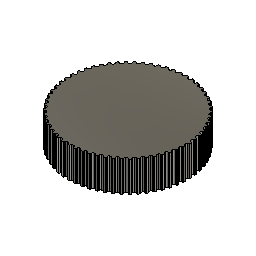
gear_62z (Autodesk Fusion 360 design; units mm, degrees)
Autodesk Fusion 360 part; units mm, degrees
sketch "Sketch1" plane through (0, 0, 0) normal (0, 0, 1) x (1, 0, 0) in component "gt2 pulley"
  circle A0 centre (0, 0) radius 19.7352 construction
  circle A1 centre (0, 0) radius 18.7312 construction
  line L0 (0, 0) -> (0, 19.7352) construction
  line L1 (0, 0) -> (0.9996, 19.7099) construction
  line L2 (0, 0) -> (1.4061, 19.6851) construction
  circle A2 centre (0, 0) radius 19.4812 construction
  arc A3 (0.3919, 19.343) -> (0.4641, 19.0491) centre (1.388, 19.4317) ccw
  circle A4 centre (0, 0) radius 19.3312 construction
  arc A5 (0.2443, 19.4797) -> (0, 19.4812) centre (0, 0) ccw
  arc A6 (0.3919, 19.343) -> (0.2443, 19.4797) centre (0.2425, 19.3297) ccw
  arc A7 (0.4641, 19.0491) -> (0.9487, 18.7072) centre (0.9768, 19.2615) ccw
  arc A8 (0, 19.4812) -> (-0.2443, 19.4797) centre (0, 0) ccw
  arc A9 (-0.2443, 19.4797) -> (-0.3919, 19.343) centre (-0.2425, 19.3297) ccw
  arc A10 (-0.4641, 19.0491) -> (-0.3919, 19.343) centre (-1.388, 19.4317) ccw
  arc A11 (-0.9486, 18.7072) -> (-0.4641, 19.0491) centre (-0.9768, 19.2615) ccw
  arc A12 (0.9487, 18.7072) -> (-0.9487, 18.7072) centre (0, 0) ccw
  point P0 (1.388, 19.4317)
  point P1 (0, 19.4812)
  dimension "d18" = 39.4704
  dimension "d19" = 2.903
  dimension "d22" = 1.004
  dimension "d24" = 0.75
  dimension "d26" = 1
  dimension "d27" = 0.15
  dimension "d28" = 0.15
  dimension "d47" = 0.555
  dimension "d52" = 3.812
  constraint coincident A0.centre A1.centre
  constraint coincident A0 L0.end
  constraint vertical L0
  constraint coincident A0 L1.end
  constraint coincident A0 L2.end
  constraint concentric A1 A2
  constraint coincident A1 A7.end
  constraint coincident L1 A7.end
  constraint coincident A2 P0
  constraint coincident L2 P0
  constraint coincident P0 A3.centre
  constraint coincident A2 P1
  constraint coincident L0 P1
  constraint concentric A2 A4
  constraint coincident P1 A5.end
  constraint coincident A4 A6.centre
  constraint coincident A3.start A6.start
  constraint tangent A3 A6
  constraint tangent A3 A7
  constraint symmetric L0 A7.end A12.end
  constraint symmetric L0 A3.start A9.end
  constraint symmetric L0 A3.end A10.start
  constraint symmetric L0 A3 A10
  constraint symmetric L0 A5.start A8.end
  constraint symmetric L0 P1 A5.end
  constraint symmetric L0 A5 A8
  constraint symmetric L0 A6 A9
  constraint symmetric L0 A7 A11
  constraint coincident A1 A11.start
  constraint tangent A1 A7
  constraint coincident L1 A7.centre
  measures "d18" diameter of A0
  measures "d19" angle of L0 L1
  measures "d22" distance of A0 A1
  measures "d24" distance of A1 A2
  measures "d26" radius of A3
  measures "d27" distance of A2 A4
  measures "d28" radius of A6
  measures "d47" radius of A7
extrude "Extrude1" add sketch "Sketch1" along normal blind 10 makes body 1
pattern_circular "C-Pattern1" count 62 over 360 about axis through (0, 0, 1.75) along (0, 0, 1) of bodies 1 makes body 2 at (-1.1593, 18.6953, 3.3333) makes body 3 at (-4.4904, 18.185, 6.6667) makes body 4 at (-5.7079, 17.8404, 6.6667) makes body 5 at (-6.7028, 17.4909, 3.3333) makes body 6 at (-8.9979, 16.4285, 6.6667) makes body 7 at (-10.7869, 15.3135, 6.6667) makes body 8 at (-12.7514, 13.7208, 6.6667) makes body 9 at (-13.0572, 13.4301, 3.3333) makes body 10 at (-15.2524, 10.8731, 6.6667) makes body 11 at (-16.2741, 9.2742, 6.6667) makes body 12 at (-17.1289, 7.5802, 6.6667) makes body 13 at (-17.2953, 7.1925, 3.3333) makes body 14 at (-18.3041, 3.977, 6.6667) makes body 15 at (-18.6126, 2.1048, 6.6667) makes body 16 at (-18.73, 0.211, 6.6667) makes body 17 at (-18.73, -0.2109, 6.6667) makes body 18 at (-18.3891, -3.5636, 6.6667) makes body 19 at (-18.3042, -3.9769, 3.3333) makes body 20 at (-17.6016, -6.4064, 6.6667) makes body 21 at (-17.1289, -7.5801, 6.6667) makes body 22 at (-15.4935, -10.5267, 6.6667) makes body 23 at (-14.7475, -11.5486, 6.6667) makes body 24 at (-14.0742, -12.3602, 3.3333) makes body 25 at (-12.1208, -14.2809, 6.6667) makes body 26 at (-10.0866, -15.7835, 6.6667) makes body 27 at (-8.998, -16.4285, 6.6667) makes body 28 at (-6.7029, -17.4908, 6.6667) makes body 29 at (-5.5068, -17.9034, 6.6667) makes body 30 at (-3.0449, -18.4821, 6.6667) makes body 31 at (-1.3699, -18.6811, 6.6667) makes body 32 at (-0.738, -18.7167, 3.3333) makes body 33 at (1.9998, -18.6242, 6.6667) makes body 34 at (4.4904, -18.185, 6.6667) makes body 35 at (6.1081, -17.7073, 6.6667) makes body 36 at (6.7028, -17.4909, 3.3333) makes body 37 at (8.9979, -16.4285, 6.6667) makes body 38 at (10.7869, -15.3135, 6.6667) makes body 39 at (12.7514, -13.7208, 6.6667) makes body 40 at (13.0572, -13.4301, 3.3333) makes body 41 at (14.8765, -11.382, 6.6667) makes body 42 at (15.9516, -9.8186, 6.6667) makes body 43 at (17.1289, -7.5802, 6.6667) makes body 44 at (17.6016, -6.4065, 6.6667) makes body 45 at (18.3041, -3.977, 6.6667) makes body 46 at (18.6126, -2.1048, 6.6667) makes body 47 at (18.73, -0.211, 6.6667) makes body 48 at (18.73, 0.2109, 3.3333) makes body 49 at (18.6126, 2.1047, 3.3333) makes body 50 at (18.3042, 3.9769, 3.3333) makes body 51 at (17.8079, 5.8083, 3.3333) makes body 52 at (16.7703, 8.3436, 6.6667) makes body 53 at (16.2742, 9.2741, 3.3333) makes body 54 at (14.349, 12.0401, 6.6667) makes body 55 at (14.0742, 12.3602, 3.3333) makes body 56 at (11.6316, 14.6821, 6.6667) makes body 57 at (10.6139, 15.4338, 6.6667) makes body 58 at (9.7285, 16.0067, 3.3333) makes body 59 at (7.4836, 17.1713, 6.6667) makes body 60 at (5.708, 17.8403, 6.6667) makes body 61 at (4.4906, 18.185, 3.3333) makes body 62 at (2.6278, 18.546, 3.3333)
sketch "Sketch2" plane through (0, 0, 10) normal (0, 0, 1) x (-1, 0, 0)
  arc A0 (-12.8969, -14.4214) -> (-12.8739, -14.6212) centre (-12.7748, -14.5086) ccw
  arc A1 (-12.8739, -14.6212) -> (-12.5031, -14.9395) centre (0, 0) ccw
  arc A2 (-12.5031, -14.9395) -> (-12.3021, -14.9319) centre (-12.4068, -14.8245) ccw
  arc A3 (-12.056, -14.756) -> (-12.3021, -14.9319) centre (-11.6041, -15.6481) ccw
  arc A4 (-11.4656, -14.8121) -> (-12.056, -14.756) centre (-11.8052, -15.2511) ccw
  arc A5 (-12.9052, -13.5762) -> (-11.4656, -14.8121) centre (0, 0) ccw
  arc A6 (-12.7602, -14.1514) -> (-12.9052, -13.5762) centre (-13.2876, -13.9785) ccw
  arc A7 (-12.8969, -14.4214) -> (-12.7602, -14.1514) centre (-13.7104, -13.8399) ccw
  circle A8 centre (0, 0) radius 18.7312
  constraint concentric A1 A8
extrude "Extrude2" add sketch "Sketch2" against normal blind 10 contours A5 A8 bodies 1 2 3 4 5 6 7 8 9 10 11 12 13 14 15 16 17 18 19 20 21 22 23 24 25 26 27 28 29 30 31 32 33 34 35 36 37 38 39 40 41 42 43 44 45 46 47 48 49 50 51 52 53 54 55 56 57 58 59 60 61 62
extrude "Extrude4" [suppressed] in component "gt2 pulley"
pattern_circular "C-Pattern7" [suppressed] in component "gt2 pulley"
extrude "Extrude3" [suppressed] in component "gt2 pulley"
pattern_circular "C-Pattern6" [suppressed] in component "gt2 pulley"
extrude "Extrude2'" [suppressed] in component "gt2 pulley"
pattern_circular "C-Pattern5" [suppressed] in component "gt2 pulley"
extrude "Extrude1'" [suppressed] in component "gt2 pulley"
pattern_circular "C-Pattern4" [suppressed] in component "gt2 pulley"
pattern_circular "C-Pattern3" [suppressed] in component "gt2 pulley"
pattern_circular "C-Pattern2" [suppressed] in component "gt2 pulley"
pattern_circular "C-Pattern1'" [suppressed] in component "gt2 pulley"
copy_body "Body->Comp1" [suppressed] in component "Component"
copy_body "Body->Comp2" [suppressed] in component "Component'"
copy_body "Body->Comp3" [suppressed] in component "Component''"
copy_body "Body->Comp4" [suppressed] in component "Component'''"
copy_body "Body->Comp5" [suppressed] in component "Component''''"
copy_body "Body->Comp6" [suppressed] in component "Component'''''"
copy_body "Body->Comp7" [suppressed] in component "Component''''''"
copy_body "Body->Comp8" [suppressed] in component "Component'''''''"
copy_body "Body->Comp9" [suppressed] in component "Component''''''''"
copy_body "Body->Comp10" [suppressed] in component "Component'''''''''"
copy_body "Body->Comp11" [suppressed] in component "Component''''''''''"
copy_body "Body->Comp12" [suppressed] in component "Component'''''''''''"
copy_body "Body->Comp13" [suppressed] in component "Component''''''''''''"
copy_body "Body->Comp14" [suppressed] in component "Component'''''''''''''"
copy_body "Body->Comp15" [suppressed] in component "Component''''''''''''''"
copy_body "Body->Comp16" [suppressed] in component "Component'''''''''''''''"
copy_body "Body->Comp17" [suppressed] in component "Component''''''''''''''''"
copy_body "Body->Comp18" [suppressed] in component "Component'''''''''''''''''"
copy_body "Body->Comp19" [suppressed] in component "Component''''''''''''''''''"
copy_body "Body->Comp20" [suppressed] in component "Component'''''''''''''''''''"
component "gt2 pulley" placed x (1, 0, 0) y (0, 1, 0) z (0, 0, 1) at (0, 0, 0)
equation "NumTeeth = 62" comment "min 20"
equation "ToothPitch = 2 mm"
equation "PullyDia = NumTeeth * ToothPitch / PI"
equation "ToothAng = ( ( 360 / NumTeeth ) * 1 deg )"
equation "TransOffsetAngle = ToothAng * 0.2"
equation "Sholulder_Radius = 0.15 mm"
equation "Root_Radius = 0.555 mm"
equation "TransRadius = 1 mm"
equation "ToolHeight = 0.75 mm"
equation "PLD = 0.254 mm"
equation "d18 = PullyDia"
equation "d19 = ToothAng / 2"
equation "d22 = PLD + ToolHeight"
equation "d24 = ToolHeight"
equation "d26 = TransRadius"
equation "d27 = Sholulder_Radius"
equation "d31 = NumTeeth"
equation "d33 = NumTeeth"
equation "d35 = NumTeeth"
equation "d37 = NumTeeth"
equation "d41 = NumTeeth"
equation "d45 = NumTeeth"
equation "d47 = Root_Radius"
equation "d50 = NumTeeth"
